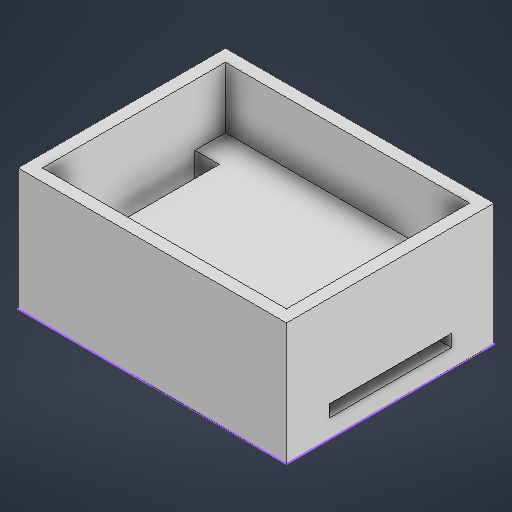
# Autodesk Inventor part: Board
Saved by Autodesk Inventor 2026.1 (Build 301233000, 233)
## iProperties
Created: 2026-07-07
Part Number: Board
Material: Generic
Document SubType Name: Modeling
Designer: Kasi Pusuluri
Density: 1 g/cm^3
Appearance: Default
Author: Kasi Pusuluri
Autodesk Inventor part; units mm, degrees
ref_plane "YZ Plane" through (0, 0, 0) normal (1, 0, 0) x (0, 1, 0)
ref_plane "XZ Plane" through (0, 0, 0) normal (0, 1, 0) x (-1, 0, 0)
ref_plane "XY Plane" through (0, 0, 0) normal (0, 0, 1) x (1, 0, 0)
sketch "Sketch1" plane through (0, 0, 0) normal (0, 1, 0) x (-1, 0, 0)
  line L0 (0, 0) -> (508, 0)
  line L1 (508, 0) -> (508, -381)
  line L2 (508, -381) -> (0, -381)
  line L3 (0, -381) -> (0, 0)
  line L4 (0, 0) -> (50.8, 0)
  line L5 (0, 0) -> (0, -12.7)
  line L6 (0, -6.35) -> (0, -57.1551)
  line L7 (0, -6.35) -> (50.8, -6.35)
  line L8 (50.8, -6.35) -> (50.8, -57.1551)
  line L9 (50.8, -57.1551) -> (0, -57.1551)
  line L10 (0, -57.1551) -> (0, -6.35)
  line L11 (0, -57.1551) -> (0, -66.0049)
  line L12 (0, -57.1551) -> (0, -69.8551)
  line L13 (0, -57.1551) -> (0, -63.5051)
  line L14 (0, -63.5051) -> (0, -317.5051)
  line L15 (0, -63.5051) -> (50.8, -63.5051)
  line L16 (50.8, -63.5051) -> (50.8, -317.5051)
  line L17 (50.8, -317.5051) -> (0, -317.5051)
  line L18 (0, -317.5051) -> (0, -63.5051)
  line L19 (0, -381) -> (0, -374.6428)
  line L20 (0, -317.5051) -> (0, -323.8478)
  line L21 (0, -323.8478) -> (50.8, -323.8478)
  line L22 (50.8, -323.8478) -> (50.8, -374.6428)
  line L23 (50.8, -374.6428) -> (0, -374.6428)
  line L24 (0, -374.6428) -> (0, -323.8478)
  line L25 (508, 0) -> (457.2, 0)
  line L26 (508, -6.35) -> (457.2, -6.35)
  line L27 (457.2, -6.35) -> (457.2, -57.1551)
  line L28 (457.2, -57.1551) -> (508, -57.1551)
  line L29 (508, -57.1551) -> (508, -6.35)
  line L30 (508, -63.5051) -> (457.2, -63.5051)
  line L31 (457.2, -63.5051) -> (457.2, -317.5051)
  line L32 (457.2, -317.5051) -> (508, -317.5051)
  line L33 (508, -317.5051) -> (508, -63.5051)
  line L34 (508, -323.8478) -> (457.2, -323.8478)
  line L35 (457.2, -323.8478) -> (457.2, -374.6428)
  line L36 (457.2, -374.6428) -> (508, -374.6428)
  line L37 (508, -374.6428) -> (508, -323.8478)
  line L38 (508, 0) -> (533.4, 0)
  line L39 (533.4, 0) -> (533.4, 25.4)
  line L40 (0, -381) -> (-25.4, -381)
  line L41 (-25.4, -381) -> (-25.4, -406.4)
  line L42 (533.4, 25.4) -> (-25.4, 25.4)
  line L43 (-25.4, 25.4) -> (-25.4, -406.4)
  line L44 (-25.4, -406.4) -> (533.4, -406.4)
  line L45 (533.4, -406.4) -> (533.4, 25.4)
  constraints: 90 end point, 15 parallel, 10 horizontal, 9 perpendicular, 7 point on line, 2 midpoint, 2 vertical, 10 other
extrude "Extrusion1" add sketch "Sketch1" along normal blind 254 contours L3 L40 L43 L42 L39 L38 L0 | L38 L45 L44 L41 L40 L2 L1
extrude "Extrusion2" add sketch "Sketch1" along normal blind 127 contours L0 L1 L26 L27 L28 L30 L31 L32 L34 L35 L36 L2 L3 L23 L22 L21 L17 L16 L15 L9 L8 L7
extrude "Extrusion3" add sketch "Sketch1" along normal blind 127 contours L7 L8 L9 L3 | L1 L28 L27 L26 | L1 L36 L35 L34 | L21 L22 L23 L3
extrude "Extrusion4" add sketch "Sketch1" along normal blind 38.1 contours L15 L16 L17 L3 | L1 L32 L31 L30
sketch "Sketch2" plane through (25.4, 0, 25.4) normal (1, 0, 0) x (0, 0, -1)
  line L0 (342.9051, 38.1) -> (88.9051, 38.1) projected
  line L1 (88.9051, 38.1) -> (88.9051, 63.5)
  line L2 (88.9051, 127) -> (88.9051, 38.1) projected
  line L3 (88.9051, 63.5) -> (342.9051, 63.5)
  line L4 (342.9051, 63.5) -> (342.9051, 38.1)
  line L5 (342.9051, 38.1) -> (88.9051, 38.1)
  line L6 (88.9051, 38.1) -> (88.9051, 63.5)
  point P0 (25.4, 0)
  dimension "d21" = 25.4
  constraints: 10 end point, 2 parallel, 1 horizontal, 1 perpendicular, 1 point on line
  measures "d21" distance of L0.end L1.end
extrude "Extrusion5" cut sketch "Sketch2" against normal blind 76.2
sketch "Sketch3" plane through (-533.4, 0, -406.4) normal (-1, 0, 0) x (0, 0, 1)
  line L0 (88.8949, 63.5) -> (88.8949, 38.1) projected
  line L1 (342.8949, 38.1) -> (342.8949, 127) projected
  line L2 (88.8949, 63.5) -> (342.8949, 63.5)
  line L3 (342.8949, 63.5) -> (342.8949, 38.1)
  line L4 (342.8949, 38.1) -> (88.8949, 38.1)
  line L5 (88.8949, 38.1) -> (88.8949, 63.5)
  point P0 (406.4, 0)
  constraints: 8 end point, 2 parallel, 1 horizontal, 1 perpendicular
extrude "Extrusion6" cut sketch "Sketch3" against normal blind 76.2
body "Solid1"
